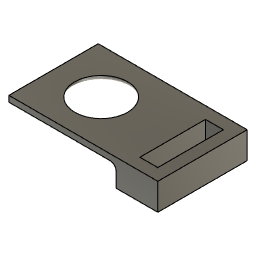
speaker mount mk1 v4 (Autodesk Fusion 360 design; units mm, degrees)
Autodesk Fusion 360 part; units mm, degrees
sketch "Sketch2" plane through (0, 0, 0) normal (0, 0, 1) x (1, 0, 0)
  line L0 (25, -15) -> (-25, -15)
  line L1 (-25, -15) -> (-25, 15)
  line L2 (-25, 15) -> (25, 15)
  line L3 (25, 15) -> (25, -15)
  line L4 (25, -15) -> (-25, 15) construction
  line L5 (-25, -15) -> (25, 15) construction
  dimension "d3" = 50
  dimension "d4" = 30
  constraint horizontal L0
  constraint perpendicular L0 L1
  constraint parallel L0 L2
  constraint parallel L1 L3
  constraint coincident L4 origin
  constraint coincident L5 origin
  measures "d3" distance of L1.end L2.end
  measures "d4" distance of L0.end L1.end
extrude "Extrude1" add sketch "Sketch2" along normal blind 2
sketch "Sketch3" plane through (0, 0, 2) normal (0, 0, 1) x (-1, 0, 0)
  line L0 (-25, -15) -> (25, -15)
  line L1 (25, -15) -> (25, 15)
  line L2 (25, 15) -> (-25, 15)
  line L3 (-25, 15) -> (-25, -15)
  circle A0 centre (9, 0) radius 8.875
  circle A1 centre (9, 0) radius 12
  dimension "d7" = 17.75
  dimension "d8" = 24
  dimension "d9" = 16
  constraint concentric A0 A1
  measures "d7" diameter of A0
  measures "d8" diameter of A1
  measures "d9" distance of L1 A0.centre
extrude "Extrude2" cut sketch "Sketch3" against normal blind 4 contours A0
sketch "Sketch4" plane through (0, 0, 0) normal (0, 0, -1) x (1, 0, 0)
  circle A0 centre (-9, 0) radius 8.875
  line L0 (-25, -15) -> (25, -15)
  line L1 (25, -15) -> (25, 15)
  line L2 (25, 15) -> (-25, 15)
  line L3 (-25, 15) -> (-25, -15)
  line L4 (25, 15) -> (11, 15)
  line L5 (11, 15) -> (11, -15)
  line L6 (11, -15) -> (25, -15)
  line L7 (25, -15) -> (25, 15)
  dimension "d12" = 14
  constraint horizontal L4
  constraint vertical L5
  constraint horizontal L6
  constraint vertical L7
  constraint coincident L0 L5.end
  constraint coincident L1.end L2.start
  measures "d12" distance of L1.end L4.end
extrude "Extrude3" add sketch "Sketch4" along normal blind 7 contours L0 L1 L2 L4 L5 L6 L7
fillet "Fillet1" radius 2 1 edges at (11, 0, 0)
fillet "Fillet2" radius 2 1 edges at (-0.7256, 3.2093, 0)
sketch "Sketch5" plane through (0, 0, -7) normal (0, 0, -1) x (1, 0, 0)
  line L0 (25, -15) -> (25, 15)
  line L1 (25, 15) -> (11, 15)
  line L2 (11, 15) -> (11, -15)
  line L3 (11, -15) -> (25, -15)
  line L4 (15, 11) -> (21, 11)
  line L5 (21, 11) -> (21, -11)
  line L6 (21, -11) -> (15, -11)
  line L7 (15, -11) -> (15, 11)
  dimension "d19" = 4
  dimension "d20" = 4
  dimension "d21" = 4
  dimension "d22" = 4
  constraint horizontal L4
  constraint vertical L5
  constraint horizontal L6
  constraint vertical L7
  measures "d19" distance of L0 L5
  measures "d20" distance of L2 L7
  measures "d21" distance of L1 L4
  measures "d22" distance of L3 L6
extrude "Extrude4" cut sketch "Sketch5" against normal blind 17 contours L4 L5 L6 L7
equation "d20 = d19"
equation "d21 = d19"
equation "d22 = d19"
